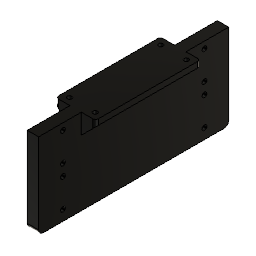
rack-nook-leg-parametric (Autodesk Fusion 360 design; units mm, degrees)
Autodesk Fusion 360 part; units mm, degrees
note: some values were not read from the file. Set by a fixed rule: the direction of a hole.
sketch "Sketch1" plane through (0, 0, 0) normal (1, 0, 0) x (0, 1, 0)
  line L0 (106, 47.625) -> (-106, 47.625)
  line L1 (-106, 47.625) -> (-106, -47.625)
  line L2 (-106, -47.625) -> (106, -47.625)
  line L3 (106, -47.625) -> (106, 47.625)
  line L4 (106, 47.625) -> (-106, -47.625) construction
  line L5 (-106, 47.625) -> (106, -47.625) construction
  line L6 (-78.88, 40.275) -> (-78.88, 8.525) construction
  line L7 (78.88, 40.275) -> (78.88, 8.525) construction
  line L8 (-78.88, 40.275) -> (78.88, 40.275) construction
  line L9 (78.88, 8.525) -> (-78.88, 8.525) construction
  line L10 (78.88, 24.4) -> (106, 24.4) construction
  line L11 (-78.88, 24.4) -> (-106, 24.4) construction
  point P0 (78.88, 8.525)
  point P1 (-78.88, 8.525)
  dimension "d390" = 212
  dimension "d391" = 95.25
  dimension "d392" = 7.35
  dimension "d5" = 31.75
  dimension "d35" = 157.76
  constraint horizontal L0
  constraint perpendicular L0 L1
  constraint parallel L0 L2
  constraint parallel L1 L3
  constraint coincident L4 origin
  constraint coincident L5 origin
  constraint coincident L7 P0
  constraint coincident L6 P1
  constraint perpendicular L0 L7
  constraint coincident P1 L6.end
  constraint coincident P0 L7.end
  constraint coincident L6.start L8.start
  constraint coincident L7.start L8.end
  constraint midpoint L7 L10.start
  constraint coincident L3 L10.end
  constraint perpendicular L3 L10
  constraint midpoint L6 L11.start
  constraint coincident L1 L11.end
  constraint perpendicular L1 L11
  constraint equal L10 L11
  constraint perpendicular L7 L9
  constraint perpendicular L7 L8
  constraint perpendicular L6 L8
  measures "d390" distance of L1.end L2.end
  measures "d391" distance of L0.end L1.end
  measures "d392" distance of L0 L6.start
  measures "d5" distance of L6.start P1
  measures "d35" distance of P1 P0
extrude "Extrude1" add sketch "Sketch1" along normal blind 12.7
hole "Hole1" at (0, -78.88, 40.275) at (0, 78.88, 40.275) at (0, -78.88, 8.525) at (0, 78.88, 8.525) direction (1, 0, 0) diameter 5.3 end up to surface (12.7 mm away)
pattern_linear "R-Pattern1" count 2 spacing 44.45 along (0, 0, -1) of "Hole1"
fillet "Fillet1" radius 5.35 2 edges at (6.35, -106, -47.625) (6.35, 106, -47.625)
sketch "Sketch2" plane through (0, 0, 47.625) normal (0, 0, 1) x (-1, 0, 0)
  line L0 (0, -106) -> (0, 106)
  line L1 (0, 106) -> (-12.7, 106)
  line L2 (-12.7, 106) -> (-12.7, -106)
  line L3 (-12.7, -106) -> (0, -106)
  line L4 (-12.7, 58.375) -> (-28.575, 58.375)
  line L5 (-28.575, 58.375) -> (-28.575, -58.375)
  line L6 (-28.575, -58.375) -> (-12.7, -58.375)
  line L7 (-12.7, -58.375) -> (-12.7, 58.375)
  dimension "d12" = 47.625
  dimension "d13" = 47.625
  dimension "d16" = 15.875
  constraint horizontal L4
  constraint vertical L5
  constraint horizontal L6
  constraint vertical L7
  constraint coincident L2 L4.start
  measures "d12" distance of L1.end L4
  measures "d13" distance of L2.end L6
  measures "d16" distance of L4.start L4.end
extrude "Extrude2" add sketch "Sketch2" against normal blind 6.35 contours L2 L4 L5 L6 L7
fillet "Fillet2" radius 3.175 2 edges at (28.575, -58.375, 44.45) (28.575, 58.375, 44.45)
chamfer "Chamfer2" distance 15.875 angle 45 1 edges at (12.7, 0, 41.275)
ref_plane "WorkPlane1" through (14.2875, 0, 41.275) normal (0, 0, 1) x (0, -1, 0)
sketch "Sketch3" plane through (0, 0, 41.275) normal (0, 0, 1) x (1, 0, 0)
  arc A0 (28.575, 55.2) -> (25.4, 58.375) centre (25.4, 55.2) ccw
  line L0 (25.4, 58.375) -> (12.7, 58.375)
  line L1 (12.7, 58.375) -> (12.7, 106)
  line L2 (12.7, 106) -> (0, 106)
  line L3 (0, 106) -> (0, -106)
  line L4 (0, -106) -> (12.7, -106)
  line L5 (12.7, -106) -> (12.7, -58.375)
  line L6 (12.7, -58.375) -> (25.4, -58.375)
  arc A1 (25.4, -58.375) -> (28.575, -55.2) centre (25.4, -55.2) ccw
  line L7 (28.575, -55.2) -> (28.575, 55.2)
  line L8 (12.7, -58.375) -> (12.7, 58.375)
  line L9 (28.575, 0) -> (12.7, 0) construction
  circle A2 centre (20.6375, -50.8) radius 5
  circle A3 centre (20.6375, 50.8) radius 5
  line L10 (20.6375, -50.8) -> (20.6375, -58.375) construction
  line L11 (20.6375, -50.8) -> (20.6375, 50.8) construction
  line L12 (20.6375, 50.8) -> (20.6375, 58.375) construction
  line L13 (20.6375, 50.8) -> (12.7, 50.8) construction
  line L14 (20.6375, 50.8) -> (28.575, 50.8) construction
  line L15 (20.6375, -50.8) -> (12.7, -50.8) construction
  line L16 (20.6375, -50.8) -> (28.575, -50.8) construction
  point P0 (20.6375, 0)
  dimension "d21" = 10
  dimension "d23" = 10
  dimension "d39" = 101.6
  constraint midpoint L7 L9.start
  constraint midpoint L8 L9.end
  constraint midpoint L9 P0
  constraint coincident A2.centre L10.start
  constraint coincident L6 L10.end
  constraint perpendicular L6 L10
  constraint coincident A3.centre L11.end
  constraint perpendicular L0 L11
  constraint perpendicular L0 L12
  constraint equal L10 L12
  constraint coincident L8 L13.end
  constraint perpendicular L8 L13
  constraint coincident L7 L14.end
  constraint perpendicular L7 L14
  constraint equal L13 L14
  constraint coincident L8 L15.end
  constraint perpendicular L8 L15
  constraint coincident L7 L16.end
  constraint perpendicular L7 L16
  constraint coincident L0 L12.end
  measures "d21" diameter of A2
  measures "d23" diameter of A3
  measures "d39" distance of A2.centre A3.centre
extrude "Extrude3" cut sketch "Sketch3" against normal blind 16 contours A2 | A3
hole "Hole2" at (20.6375, -50.8, 41.275) at (20.6375, 50.8, 41.275) direction (0, 0, 1) diameter 5 end up to surface (6.35 mm away)
ref_plane "WorkPlane2" through (6.35, 0, 0) normal (1, 0, 0) x (0, 0, -1)
mirror "Mirror1" about plane through (6.35, 0, 0) normal (1, 0, 0) of bodies 1 merged
equation "d390 = RackDepth + LegFrontSpacing + LegBackSpacing"
equation "d391 = 1.75 \" * RackUnits + LegTopSpacing + LegBottomSpacing"
equation "d392 = 1/4\" + LegTopSpacing"
equation "d396 = 21.40 mm + 4 mm"
equation "d402 = LegWidth"
equation "LegHeight = ( 1.75 \" * RackUnits ) + LegTopSpacing + LegBottomSpacing"
equation "LegWidth = 0.5 \""
equation "RackUnits = 2"
equation "LegTopSpacing = 1 mm"
equation "LegBottomSpacing = 1/4\" - LegTopSpacing"
equation "d2 = 1/4\" - 1 mm"
equation "d5 = 1.25 \""
equation "d12 = 1 7/8\""
equation "d13 = d12"
equation "d14 = -1/4\""
equation "d16 = 5/8\""
equation "d18 = 1/8\""
equation "d19 = 5/8\""
equation "d20 = -1/4\""
equation "d31 = RackUnits"
equation "d33 = 1.75 \""
equation "d35 = RackDepth - 42.24 mm"
equation "RackDepth = 200 mm"
equation "LegFrontSpacing = 6 mm"
equation "LegBackSpacing = 6 mm"
equation "d39 = 4\""
